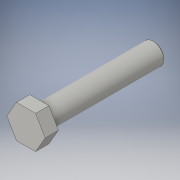
# Autodesk Inventor part: 1.5in bolt
Saved by Autodesk Inventor 2016 (Build 200138000, 138)
## iProperties
Created: 2015-10-31
Part Number: 1.5in bolt
Material: Generic
Document SubType Name: Modeling
Designer: Delta
Density: 1 g/cm^3
Appearance: Default
Author: Delta
Autodesk Inventor part; units mm, degrees
ref_plane "YZ Plane" through (0, 0, 0) normal (1, 0, 0) x (0, 1, 0)
ref_plane "XZ Plane" through (0, 0, 0) normal (0, 1, 0) x (-1, 0, 0)
ref_plane "XY Plane" through (0, 0, 0) normal (0, 0, 1) x (1, 0, 0)
sketch "Sketch1" plane through (0, 0, 0) normal (0, 0, 1) x (1, 0, 0)
  circle A0 centre (0, 0) radius 3.175
  dimension "d0" = 6.35
  constraints: 1 centre point, 1 coincident
  measures "d0" diameter of A0
extrude "Extrusion1" add sketch "Sketch1" along normal blind 38.1
sketch "Sketch2" plane through (0, 0, 38.1) normal (0, 0, 1) x (1, 0, 0)
  line L0 (5.693, 0) -> (2.8465, -4.9303)
  line L1 (2.8465, -4.9303) -> (-2.8465, -4.9303)
  line L2 (-2.8465, -4.9303) -> (-5.693, 0)
  line L3 (-5.693, 0) -> (-2.8465, 4.9303)
  line L4 (-2.8465, 4.9303) -> (2.8465, 4.9303)
  line L5 (2.8465, 4.9303) -> (5.693, 0)
  point P0 (0, 0)
  point P1 (0, 0)
  constraints: 12 end point, 1 coincident, 13 other
extrude "Extrusion2" add sketch "Sketch2" against normal blind 3.9688
chamfer "Chamfer1" distance 0.254 angle 45 1 edges at (-3.175, 0, 0)
body "Solid1"
